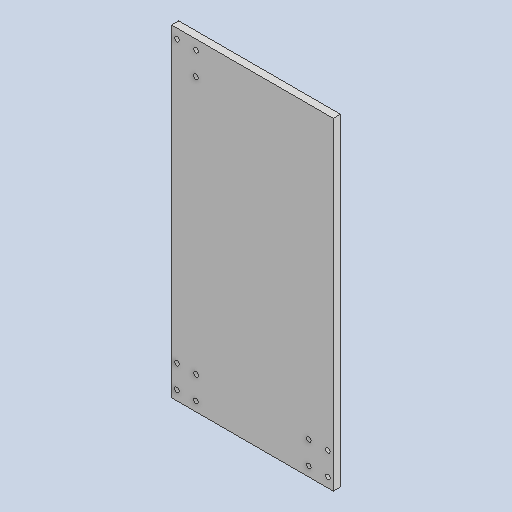
# Autodesk Inventor part: base
Saved by Autodesk Inventor 2022 (Build 260153000, 153)
## iProperties
Created: 2023-05-18
Part Number: base
Material: Типовые
Document SubType Name: Modeling
Designer: Robo0
Density: 1 g/cm^3
Appearance: По умолчанию
Author: Robo0
Autodesk Inventor part; units mm, degrees
ref_plane "YZ Plane" through (0, 0, 0) normal (1, 0, 0) x (0, 1, 0)
ref_plane "XZ Plane" through (0, 0, 0) normal (0, 1, 0) x (-1, 0, 0)
ref_plane "XY Plane" through (0, 0, 0) normal (0, 0, 1) x (1, 0, 0)
sketch "Эскиз1" plane through (0, 0, 0) normal (0, 0, 1) x (1, 0, 0)
  circle A0 centre (-29.5, -29.7047) radius 2 projected
  circle A1 centre (-45.5, -29.7047) radius 2 projected
  circle A2 centre (-45.5, -10.2953) radius 2 projected
  circle A3 centre (-29.5, -10.2953) radius 2 projected
  circle A4 centre (-156.1512, -29.6896) radius 2 projected
  circle A5 centre (-140.1512, -29.6896) radius 2 projected
  circle A6 centre (-140.1512, -10.2803) radius 2 projected
  circle A7 centre (-156.1512, -10.2803) radius 2 projected
  circle A8 centre (-140.1512, 205.7348) radius 2 projected
  circle A9 centre (-156.1512, 205.7348) radius 2 projected
  circle A10 centre (-140.1512, 225.1441) radius 2 projected
  circle A11 centre (-156.1512, 225.1441) radius 2 projected
  circle A12 centre (-29.5, 225.129) radius 2 projected
  circle A13 centre (-29.5, 205.7197) radius 2 projected
  circle A14 centre (-45.5, 205.7197) radius 2 projected
  circle A15 centre (-45.5, 225.129) radius 2 projected
  line L0 (-25, -41.891) -> (-25, 1.891) projected
  line L1 (-11.2, 1) -> (-52.2, 1)
  line L2 (-160.6512, 237.3305) -> (-160.6512, 193.5485) projected
  line L3 (-132.8256, 233.1441) -> (-185.6512, 233.1441) projected
  line L4 (-52.8256, -37.7047) -> (0, -37.7047) projected
  line L5 (-25, -37.7047) -> (-160.6512, -37.7047)
  line L6 (-160.6512, -37.7047) -> (-160.6512, 233.1441)
  line L7 (-160.6512, 233.1441) -> (-25, 233.1441)
  line L8 (-25, 233.1441) -> (-25, -37.7047)
  point P0 (0, 0)
  point P1 (-160.6512, 187.3305)
  point P2 (-25, -21.891)
  constraints: 10 end point, 4 point on line, 2 horizontal, 2 parallel, 1 perpendicular, 2 other
extrude "Выдавливание1" add sketch "Эскиз1" along normal blind 6 contours A9 | A12 | A13 | A14 | A15 | L4 L5 L6 L2 L3 L7 L8 L0
